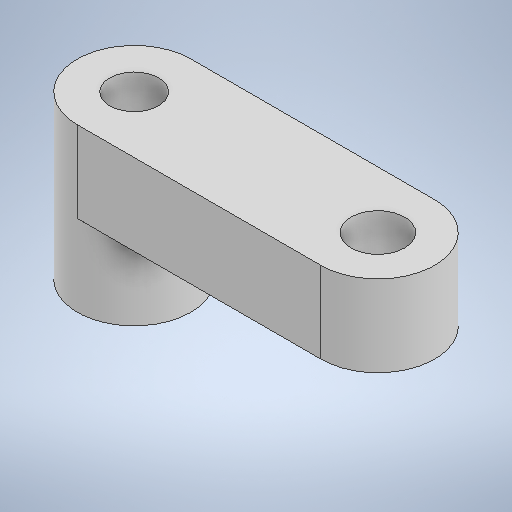
# Autodesk Inventor part: m
Saved by Autodesk Inventor 2026 (Build 300175050, 175E)
## iProperties
Created: 2025-05-24
Part Number: m
Material: Generic
Document SubType Name: Modeling
Designer: omiye
Density: 1 g/cm^3
Appearance: Default
Author: omiye
Autodesk Inventor part; units mm, degrees
ref_plane "YZ Plane" through (0, 0, 0) normal (1, 0, 0) x (0, 1, 0)
ref_plane "XZ Plane" through (0, 0, 0) normal (0, 1, 0) x (-1, 0, 0)
ref_plane "XY Plane" through (0, 0, 0) normal (0, 0, 1) x (1, 0, 0)
sketch "Sketch1" plane through (0, 0, 0) normal (0, 1, 0) x (-1, 0, 0)
  line L0 (-7.5, -3.5) -> (-7.5, 3.5)
  line L1 (-7.5, 3.5) -> (7.5, 3.5)
  line L2 (7.5, 3.5) -> (7.5, -3.5)
  line L3 (7.5, -3.5) -> (-7.5, -3.5)
  line L4 (-7.5, -3.5) -> (7.5, 3.5) construction
  line L5 (-7.5, 3.5) -> (7.5, -3.5) construction
  circle A0 centre (7.5, 0) radius 1.5
  circle A1 centre (-7.5, 0) radius 1.65
  line L6 (7.5, 3.5) -> (11, 3.5)
  line L7 (11, 3.5) -> (11, -3.5)
  line L8 (11, -3.5) -> (7.5, -3.5)
  line L9 (7.5, -3.5) -> (7.5, 3.5)
  line L10 (-7.5, 3.5) -> (-11, 3.5)
  line L11 (-11, 3.5) -> (-11, -3.5)
  line L12 (-11, -3.5) -> (-7.5, -3.5)
  line L13 (-7.5, -3.5) -> (-7.5, 3.5)
  point P0 (0, 0)
  dimension "d0" = 7
  dimension "d1" = 15
  dimension "d2" = 3
  dimension "d3" = 3.3
  dimension "d4" = 3.5
  dimension "d5" = 3.5
  constraints: 28 end point, 6 parallel, 4 midpoint, 3 perpendicular, 2 centre point, 2 horizontal, 1 point on line, 1 vertical
  measures "d0" distance of L0.start L0.end
  measures "d1" distance of L0.end L1.end
  measures "d2" diameter of A0
  measures "d3" diameter of A1
  measures "d4" distance of L7.end L8.end
  measures "d5" distance of L12.end L11.end
extrude "Extrusion1" add sketch "Sketch1" along normal blind 5 contours L12 L11 L10 L0 A1 | L0 A1 L1 L2 A0 L3 | L2 A0 L6 L7 L8
fillet "Fillet1" radius 3.5 4 edges at (-11, 2.5, -3.5) (-11, 2.5, 3.5) (11, 2.5, 3.5) (11, 2.5, -3.5)
sketch "Sketch2" plane through (0, 0, 0) normal (0, -1, 0) x (1, 0, 0)
  circle A0 centre (-7.5, 0) radius 1.5 projected
  circle A1 centre (-7.5, 0) radius 3.5
  circle A2 centre (-7.5, 0) radius 1.65
  point P0 (0, 0)
  dimension "d9" = 3.3
  constraints: 2 centre point, 2 coincident
  measures "d9" diameter of A2
extrude "Extrusion2" add sketch "Sketch2" along normal blind 5 contours A1 | A2
body "Solid1"
